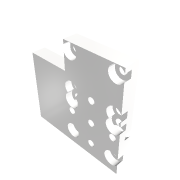
# Autodesk Inventor part: Gripper_linear_arm_1
Saved by Autodesk Inventor 2022 (Build 260153000, 153)
## iProperties
Created: 2023-01-05
Part Number: Gripper_linear_arm_1
Material: Generisch
Document SubType Name: Modeling
Designer: diederichbenedict
Density: 1 g/cm^3
Appearance: Glatt - Weiß
Author: diederichbenedict
Autodesk Inventor part; units mm, degrees
ref_plane "YZ Plane" through (0, 0, 0) normal (1, 0, 0) x (0, 1, 0)
ref_plane "XZ Plane" through (0, 0, 0) normal (0, 1, 0) x (-1, 0, 0)
ref_plane "XY Plane" through (0, 0, 0) normal (0, 0, 1) x (1, 0, 0)
ref_plane "Arbeitsebene1" through (-19.3, 0, 0) normal (0, 0, 1) x (1, 0, 0)
sketch "Skizze1" plane through (-19.3, 0, 0) normal (0, 0, 1) x (1, 0, 0)
  line L0 (19.3, -32.4) -> (25.8, -32.4) projected
  line L1 (25.8, 0) -> (25.8, -32.4) projected
  line L2 (19.3, 0) -> (25.8, 0) projected
  line L3 (19.3, 0) -> (19.3, -32.4) projected
  circle A0 centre (22.9, -6.2) radius 1.75 projected
  circle A1 centre (22.9, -26.2) radius 1.75 projected
  line L4 (0, -32.4) -> (6.5, -32.4) projected
  line L5 (6.5, 0) -> (6.5, -32.4) projected
  line L6 (0, 0) -> (6.5, 0) projected
  line L7 (0, 0) -> (0, -32.4) projected
  circle A2 centre (2.9, -6.2) radius 1.75 projected
  circle A3 centre (2.9, -26.2) radius 1.75 projected
  line L8 (25.8, 0) -> (-19.2, 0)
  line L9 (-19.2, 0) -> (-19.2, -32.4)
  line L10 (-19.2, -32.4) -> (25.8, -32.4)
  line L11 (25.8, -32.4) -> (25.8, 0)
  dimension "d0" = 45
  constraints: 8 end point, 2 parallel, 1 horizontal, 1 perpendicular
  measures "d0" distance of L10.end L9.end
extrude "Extrusion1" add sketch "Skizze1" along normal blind 6
sketch "Skizze2" plane through (-38.5, -32.4, 0) normal (0, -1, 0) x (1, 0, 0)
  circle A0 centre (5.95, -6) radius 1.75 projected
  line L0 (0, 0) -> (45, 0) projected
  line L1 (45, 0) -> (45, 6) projected
  line L2 (0, 6) -> (45, 6) projected
  line L3 (0, 0) -> (0, 6) projected
  line L4 (45, 0) -> (0, 0) projected
  line L5 (0, 0) -> (12, 0)
  line L6 (12, 0) -> (12, -12)
  line L7 (12, -12) -> (0, -12)
  line L8 (0, -12) -> (0, 0)
  circle A1 centre (5.95, -6) radius 1.6
  point P0 (38.5, 0)
  dimension "d3" = 12
  dimension "d4" = 12
  dimension "d5" = 3.2
  constraints: 8 end point, 2 parallel, 1 centre point, 1 coincident, 1 horizontal, 1 perpendicular
  measures "d3" distance of L6.end L7.end
  measures "d4" distance of L5.end L6.end
  measures "d5" diameter of A1
extrude "Extrusion2" add sketch "Skizze2" against normal blind 6 contours L0 L6 L7 L8
sketch "Skizze3" plane through (-19.3, 0, 6) normal (0, 0, 1) x (1, 0, 0)
  circle A0 centre (22.9, -6.2) radius 1.75 projected
  circle A1 centre (22.9, -26.2) radius 1.75 projected
  circle A2 centre (2.9, -26.2) radius 1.75 projected
  circle A3 centre (2.9, -6.2) radius 1.75 projected
  point P0 (19.3, 0)
hole "Bohrung1" at (3.6, -26.2, 6) at (3.6, -6.2, 6) at (-16.4, -6.2, 6) at (-16.4, -26.2, 6) direction (0, 0, -1) diameter 3 end through all counterbore diameter 6.5 counterbore depth 3
sketch "Skizze4" plane through (-19.3, 0, 0) normal (0, 0, 1) x (1, 0, 0)
  arc A0 (25.8, -24.7328) -> (25.8, -27.6672) centre (22.9, -26.2) ccw projected
  line L0 (25.8, -24.7328) -> (25.8, -7.6672) projected
  arc A1 (25.8, -4.7328) -> (25.8, -7.6672) centre (22.9, -6.2) ccw projected
  line L1 (25.8, -4.7328) -> (25.8, 0) projected
  line L2 (25.8, 0) -> (-19.2, 0) projected
  line L3 (-19.2, 0) -> (-19.2, -32.4) projected
  line L4 (-19.2, -32.4) -> (25.8, -32.4) projected
  line L5 (25.8, -32.4) -> (25.8, -27.6672) projected
  circle A2 centre (2.9, -26.2) radius 3.25 projected
  circle A3 centre (2.9, -6.2) radius 3.25 projected
  circle A4 centre (22.9, -16.2) radius 1.4
  circle A5 centre (2.9, -16.2) radius 1.4
  circle A6 centre (12.9, -16.2) radius 1.4
  circle A7 centre (12.9, -6.2) radius 1.4
  circle A8 centre (12.9, -26.2) radius 1.4
  point P0 (19.3, 0)
  dimension "d15" = 2.8
  dimension "d16" = 2.8
  dimension "d17" = 20
  dimension "d18" = 0
  dimension "d19" = 2.8
  dimension "d20" = 10
  dimension "d21" = 2.8
  dimension "d22" = 2.8
  constraints: 5 centre point, 5 coincident
  measures "d15" diameter of A4
  measures "d16" diameter of A5
  measures "d17" distance of A5.centre A4.centre
  measures "d18" horizontal distance of A0.centre A4.centre
  measures "d19" diameter of A6
  measures "d20" horizontal distance of A6.centre A0.centre
  measures "d21" diameter of A7
  measures "d22" diameter of A8
hole "Bohrung2" at (-16.4, -16.2, 0) at (-6.4, -16.2, 0) at (-6.4, -26.2, 0) at (3.6, -16.2, 0) at (-6.4, -6.2, 0) direction (0, 0, 1) diameter 3 end through all counterbore diameter 6.5 counterbore depth 3
sketch "Skizze5" plane through (-38.5, -26.4, 0) normal (0, 1, 0) x (1, 0, 0)
  point P0 (38.5, 0)
sketch "Skizze6" plane through (-38.5, -32.4, 6) normal (0, -1, 0) x (1, 0, 0)
  circle A0 centre (5.95, -12) radius 1.75 projected
  circle A1 centre (5.95, -12) radius 3.5
  point P0 (38.5, -6)
  dimension "d30" = 7
  constraints: 1 centre point, 1 coincident
  measures "d30" diameter of A1
extrude "Extrusion3" cut sketch "Skizze6" against normal blind 4 contours A0 | A1
sketch "Skizze7" plane through (-19.3, 0, 6) normal (0, 0, 1) x (1, 0, 0)
  line L0 (25.8, -4.7328) -> (25.8, 0) projected
  circle A0 centre (22.9, -16.2) radius 1.5 projected
  circle A1 centre (12.9, -16.2) radius 1.5 projected
  circle A2 centre (2.9, -16.2) radius 1.5 projected
  circle A3 centre (12.9, -26.2) radius 1.5 projected
  circle A4 centre (12.9, -6.2) radius 1.5 projected
  arc A5 (25.8, -24.7328) -> (25.8, -27.6672) centre (22.9, -26.2) ccw projected
  line L1 (25.8, -24.7328) -> (25.8, -7.6672) projected
  arc A6 (25.8, -4.7328) -> (25.8, -7.6672) centre (22.9, -6.2) ccw projected
  line L2 (25.8, -4.7328) -> (25.8, 0) projected
  line L3 (25.8, 0) -> (-19.2, 0) projected
  line L4 (-19.2, 0) -> (-19.2, -32.4) projected
  line L5 (-19.2, -32.4) -> (25.8, -32.4) projected
  line L6 (25.8, -32.4) -> (25.8, -27.6672) projected
  circle A7 centre (2.9, -26.2) radius 3.25 projected
  circle A8 centre (2.9, -6.2) radius 3.25 projected
  line L7 (0, 0) -> (0, -32.4) projected
  line L8 (25.8, 0) -> (0, 0)
  line L9 (0, 0) -> (0, 12)
  line L10 (0, 12) -> (25.8, 12)
  line L11 (25.8, 12) -> (25.8, 0)
  point P0 (19.3, 0)
  dimension "d34" = 12
  constraints: 8 end point, 2 parallel, 1 horizontal, 1 perpendicular
  measures "d34" distance of L7.start L9.end
extrude "Extrusion4" add sketch "Skizze7" against normal blind 6 contours L3 L9 L10 L11
sketch "Skizze8" plane through (-19.3, 0, 6) normal (0, 0, 1) x (1, 0, 0)
  circle A0 centre (22.9, 8.6709) radius 1.75
  circle A1 centre (2.9, 8.6709) radius 1.75
  circle A2 centre (22.9, -11.3291) radius 1.75
  circle A3 centre (2.9, -11.3291) radius 1.5
  line L0 (-3.15, 35.6) -> (-3.15, -57.8)
  point P0 (19.3, 14.8709)
  constraints: 4 centre point, 2 end point
hole "Bohrung3" at (3.6, 8.6709, 6) at (3.6, -11.3291, 6) at (-16.4, 8.6709, 6) at (-16.4, -11.3291, 6) direction (0, 0, -1) diameter 3 end through all counterbore diameter 6.5 counterbore depth 3
